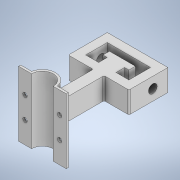
# Autodesk Inventor part: Clamp jaw
Saved by Autodesk Inventor 2022 (Build 260153000, 153)
## iProperties
Created: 2021-06-24
Part Number: Clamp jaw
Material: Generic
Document SubType Name: Modeling
Designer: Admin
Density: 1 g/cm^3
Appearance: Default
Author: Admin
Autodesk Inventor part; units mm, degrees
ref_plane "YZ Plane" through (0, 0, 0) normal (1, 0, 0) x (0, 1, 0)
ref_plane "XZ Plane" through (0, 0, 0) normal (0, 1, 0) x (-1, 0, 0)
sketch "Sketch1" plane through (0, 0, 0) normal (0, 1, 0) x (-1, 0, 0)
  arc A0 (-25, 0) -> (25, 0) centre (0, 0) ccw
  arc A1 (-29.5804, -5) -> (29.5804, -5) centre (0, 0) ccw
  line L0 (25, 0) -> (55, 0)
  line L1 (55, 0) -> (55, -5)
  line L2 (55, -5) -> (29.5804, -5)
  line L3 (-25, 0) -> (-45, 0)
  line L4 (-45, -5) -> (-29.5804, -5)
  line L5 (0, 0) -> (12.5, 0) construction
  line L6 (12.5, -300) -> (0, -300) construction
  line L7 (0, -185) -> (0, 0) construction
  line L8 (0, 0) -> (-12.5, 0) construction
  line L9 (-12.5, -300) -> (0, -300) construction
  line L10 (0, 0) -> (0, -150) construction
  line L11 (-40, -150) -> (40, -150)
  line L12 (40, -160) -> (40, -210)
  line L13 (-30, -210) -> (-40, -210) construction
  line L14 (-40, -210) -> (-40, -160)
  line L15 (-40, -150) -> (40, -210) construction
  line L16 (40, -150) -> (-40, -210) construction
  line L17 (40, -150) -> (50, -150)
  line L18 (50, -150) -> (50, -210)
  line L19 (50, -210) -> (40, -210)
  line L20 (-40, -150) -> (-50, -150)
  line L21 (-50, -150) -> (-50, -210)
  line L22 (-50, -210) -> (-40, -210)
  line L23 (12.5, -150) -> (12.5, -160) construction
  line L24 (12.5, -150) -> (12.5, -160)
  line L25 (40, -160) -> (12.5, -160)
  line L26 (-12.5, -160) -> (-40, -160)
  line L27 (0, -160) -> (20, -160) construction
  line L28 (20, -160) -> (20, -170)
  line L29 (20, -170) -> (30, -170)
  line L30 (30, -170) -> (30, -185)
  line L31 (30, -185) -> (0, -185)
  line L32 (0, -160) -> (-20, -160) construction
  line L33 (-20, -160) -> (-20, -170)
  line L34 (-20, -170) -> (-30, -170)
  line L35 (-30, -170) -> (-30, -185)
  line L36 (-30, -185) -> (0, -185)
  line L37 (-25, 0) -> (-55, 0)
  line L38 (-55, -5) -> (-29.5804, -5)
  line L39 (-55, 0) -> (-55, -5)
  line L40 (12.5, -27.2718) -> (12.5, -150)
  line L41 (-12.5, -27.2718) -> (-12.5, -150)
  point P0 (0, -180)
  dimension "d0" = 50
  dimension "d1" = 60
  dimension "d2" = 30
  dimension "d3" = 5
  dimension "d5" = 5
  dimension "d6" = 12.5
  dimension "d7" = 300
  dimension "d8" = 150
  dimension "d9" = 80
  dimension "d10" = 60
  dimension "d11" = 10
  dimension "d12" = 10
  dimension "d13" = 20
  dimension "d14" = 10
  dimension "d15" = 10
  dimension "d16" = 15
  constraints: 84 end point, 12 point on line, 10 perpendicular, 10 symmetric about line, 6 point on circle, 5 horizontal, 4 parallel, 2 centre point, 2 coincident, 2 midpoint, 1 collinear
  measures "d0" diameter of A0
  measures "d1" diameter of A1
  measures "d2" distance of L0.start L0.end
  measures "d3" distance of L0.end L1.end
  measures "d5" distance of L3.end L4.start
  measures "d6" distance of L6.start L6.end
  measures "d7" distance of L5.end L6.start
  measures "d8" distance of L5.start L10.end
  measures "d9" distance of L12.end L13.end
  measures "d10" distance of L11.end L12.end
  measures "d11" distance of L11.end L17.end
  measures "d12" distance of L23.end L23.start
  measures "d13" distance of L27.start L27.end
  measures "d14" distance of L27.end L28.end
  measures "d15" distance of L28.end L29.end
  measures "d16" distance of L29.end L30.end
extrude "Extrusion1" add sketch "Sketch1" along normal blind 150 contours A0 L0 L1 L2 A1 L4 L38 L39 L37 L3
ref_plane "Work Plane1" through (0, 75, 0) normal (0, 1, 0) x (1, 0, 0)
sketch "Sketch3" plane through (0, 75, 0) normal (0, 1, 0) x (1, 0, 0)
  line L0 (25, 0) -> (55, 0)
  line L1 (-25, 0) -> (-45, 0)
  line L2 (0, 0) -> (12.5, 0) construction
  line L3 (0, 0) -> (-12.5, 0) construction
  line L4 (-25, 0) -> (-55, 0)
  arc A0 (25, 0) -> (-25, 0) centre (0, 0) ccw
  arc A1 (29.5804, 5) -> (-29.5804, 5) centre (0, 0) ccw
  line L5 (55, 0) -> (55, 5)
  line L6 (55, 5) -> (29.5804, 5)
  line L7 (-45, 5) -> (-29.5804, 5)
  line L8 (0, 185) -> (0, 0) construction
  line L9 (0, 0) -> (0, 150) construction
  line L10 (-40, 150) -> (40, 210) construction
  line L11 (40, 150) -> (-40, 210) construction
  line L12 (40, 150) -> (50, 150)
  line L13 (50, 150) -> (50, 200)
  line L14 (-50, 150) -> (-50, 200)
  line L15 (-40, 150) -> (-50, 150)
  line L16 (0, 160) -> (12.5, 160) construction
  line L17 (20, 160) -> (20, 170)
  line L18 (20, 170) -> (30, 170)
  line L19 (30, 170) -> (30, 185)
  line L20 (30, 185) -> (0, 185)
  line L21 (0, 160) -> (-12.5, 160) construction
  line L22 (-20, 160) -> (-20, 170)
  line L23 (-20, 170) -> (-30, 170)
  line L24 (-30, 170) -> (-30, 185)
  line L25 (-30, 185) -> (0, 185)
  line L26 (-55, 5) -> (-29.5804, 5)
  line L27 (12.5, 27.2718) -> (12.5, 130)
  line L28 (-12.5, 27.2718) -> (-12.5, 130)
  line L29 (-40, 150) -> (-20, 150)
  line L30 (20, 150) -> (40, 150)
  line L31 (-70, 200) -> (-70, 140)
  line L32 (50, 150) -> (50, 200)
  line L33 (-50, 200) -> (-50, 150)
  line L34 (-50, 150) -> (50, 210) construction
  line L35 (50, 150) -> (-50, 210) construction
  line L36 (20, 160) -> (20, 150)
  line L37 (-20, 160) -> (-20, 150)
  line L38 (-50, 150) -> (-20, 150)
  line L39 (20, 150) -> (50, 150)
  line L40 (70, 200) -> (70, 140)
  line L41 (-50, 150) -> (50, 150)
  line L42 (50, 150) -> (50, 200)
  line L43 (-50, 200) -> (-50, 150)
  line L44 (-70, 140) -> (-70, 130)
  line L45 (-70, 130) -> (-12.5, 130)
  line L46 (12.5, 130) -> (70, 130)
  line L47 (70, 130) -> (70, 140)
  line L48 (-50, 200) -> (50, 200)
  line L49 (70, 200) -> (70, 220)
  line L50 (70, 220) -> (-70, 220)
  line L51 (-70, 220) -> (-70, 200)
  point P0 (-45, -5)
  point P1 (0, 180)
  dimension "d21" = 30
  dimension "d62" = 50
  dimension "d63" = 10
  dimension "d65" = 20
  constraints: 104 end point, 7 horizontal, 6 parallel, 6 perpendicular, 6 point on circle, 6 point on line, 4 coincident, 4 midpoint, 2 centre point, 1 vertical
  measures "d21" distance of L0.start L0.end
  measures "d62" distance of L13.end L41.end
  measures "d63" distance of L31.end L44.end
  measures "d65" distance of L49.end L49.start
extrude "Extrusion2" add sketch "Sketch3" along normal mid plane 50 contours A1 L28 L45 L44 L31 L51 L50 L49 L40 L47 L46 L27 | L41 L37 L22 L23 L24 L25 L20 L19 L18 L17 L36
sketch "Sketch5" plane through (-50, 50, -150) normal (1, 0, 0) x (0, 0, 1)
  line L0 (-35, 0) -> (-35, -50) construction
  circle A0 centre (-35, -25) radius 10
  point P0 (150, 50)
  dimension "d38" = 20
  constraints: 1 centre point, 1 midpoint
  measures "d38" diameter of A0
extrude "Extrusion4" cut sketch "Sketch5" against normal blind 20
sketch "Sketch6" plane through (55, 0, -5) normal (0, 0, -1) x (-1, 0, 0)
  line L0 (30, 0) -> (0, 0) projected
  line L1 (15, 0) -> (15, 50) construction
  line L2 (15, 50) -> (15, 100) construction
  circle A0 centre (15, 100) radius 5
  circle A1 centre (15, 50) radius 5
  point P0 (55, 0)
  dimension "d43" = 50
  dimension "d44" = 50
  dimension "d45" = 10
  dimension "d46" = 10
  constraints: 4 end point, 2 centre point, 2 coincident, 1 midpoint, 1 point on line, 1 vertical
  measures "d43" distance of L1.start L1.end
  measures "d44" distance of L1.end L2.end
  measures "d45" diameter of A0
  measures "d46" diameter of A1
extrude "Extrusion5" cut sketch "Sketch6" against normal blind 10
sketch "Sketch7" plane through (-29.5804, 0, -5) normal (0, 0, -1) x (-1, 0, 0)
  line L0 (25.4196, 0) -> (-4.5804, 0) projected
  line L1 (10.4196, 50) -> (10.4196, 100) construction
  line L2 (10.4196, 0) -> (10.4196, 50) construction
  line L3 (10.4196, 50) -> (10.4196, 100)
  circle A0 centre (10.4196, 100) radius 5
  circle A1 centre (10.4196, 50) radius 5
  point P0 (-29.5804, 0)
  dimension "d49" = 50
  dimension "d50" = 50
  dimension "d51" = 10
  dimension "d52" = 10
  constraints: 4 end point, 2 centre point, 2 coincident, 1 collinear, 1 midpoint, 1 vertical
  measures "d49" distance of L2.start L1.start
  measures "d50" distance of L1.start L1.end
  measures "d51" diameter of A0
  measures "d52" diameter of A1
extrude "Extrusion6" cut sketch "Sketch7" against normal blind 10
fillet "Fillet2" radius 3 4 edges at (70, 75, -130) (12.5, 75, -130) (-12.5, 75, -130) (-70, 75, -130)
sketch "Sketch8" plane through (70, 50, -220) normal (1, 0, 0) x (0, 0, -1)
  line L0 (-35, 0) -> (-35, 50) projected
  circle A0 centre (-35, 25) radius 10
  point P0 (-220, -50)
  dimension "d66" = 20
  constraints: 1 centre point, 1 midpoint
  measures "d66" diameter of A0
extrude "Extrusion7" cut sketch "Sketch8" against normal blind 20
thread "Thread1" size "M20x2.5" class "6H" standard "ANSI Metric M Profile" full length
body "Solid1"
